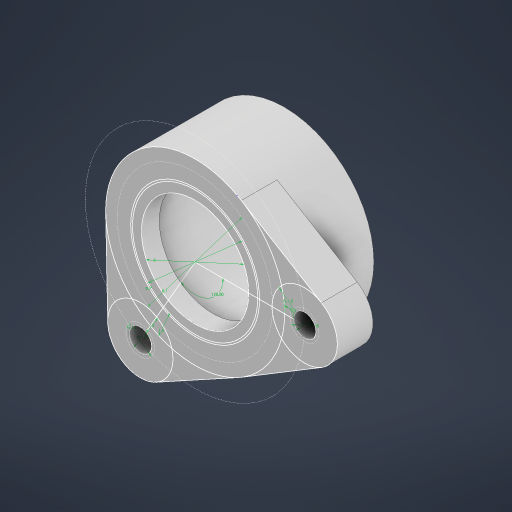
# Autodesk Inventor part: encoderauxiliary
Saved by Autodesk Inventor 2023.5 (Build 275446000, 446)
## iProperties
Created: 2024-12-07
Part Number: encoderauxiliary
Material: 一般
Document SubType Name: Modeling
Designer: IshiiLabHonda
Density: 1 g/cm^3
Appearance: 既定
Author: IshiiLabHonda
Autodesk Inventor part; units mm, degrees
ref_plane "YZ Plane" through (0, 0, 0) normal (1, 0, 0) x (0, 1, 0)
ref_plane "XZ Plane" through (0, 0, 0) normal (0, 1, 0) x (-1, 0, 0)
ref_plane "XY Plane" through (0, 0, 0) normal (0, 0, 1) x (1, 0, 0)
sketch "スケッチ1" plane through (0, 0, 0) normal (0, 0, 1) x (1, 0, 0)
  circle A0 centre (0, 0) radius 4.35 construction
  circle A1 centre (0, 0) radius 3.6
  circle A2 centre (0, 0) radius 5
  circle A3 centre (0, 0) radius 6.125 construction
  circle A4 centre (-3.0625, -5.3044) radius 0.625
  circle A5 centre (6.125, 0) radius 0.625
  circle A6 centre (-3.0625, -5.3044) radius 1.825
  circle A7 centre (6.125, 0) radius 1.825
  circle A8 centre (6.125, 0) radius 0.8 construction
  circle A9 centre (-3.0625, -5.3044) radius 0.8 construction
  line L0 (-4.9989, -0.1067) -> (-4.8871, -5.3434)
  line L1 (-2.1839, -6.904) -> (2.407, -4.3825)
  line L2 (2.5918, -4.2758) -> (7.071, -1.5607)
  line L3 (7.071, 1.5607) -> (2.5918, 4.2758)
  circle A10 centre (0, 0) radius 3
  line L4 (0, 0) -> (-3.0625, -5.3044)
  line L5 (0, 0) -> (6.125, 0)
  circle A11 centre (0, 0) radius 3.5
  point P0 (2.3702, 4.4025)
  dimension "d0" = 8.7
  dimension "d3" = 1.25
  dimension "d4" = 1.25
  dimension "d5" = 1.2
  dimension "d6" = 1.2
  dimension "d7" = 0.5
  dimension "d8" = 1.6
  dimension "d9" = 1.6
  dimension "d14" = 6
  dimension "d19" = 120
  dimension "d26" = 0.1
  dimension "d27" = 7
  dimension "d28" = 1.5
  constraints: 12 centre point, 12 end point, 11 coincident, 11 point on circle, 8 tangent, 1 horizontal
  measures "d0" diameter of A0
  measures "d3" diameter of A4
  measures "d4" diameter of A5
  measures "d5" radial gap between concentric circles of A4 A6
  measures "d6" radial gap between concentric circles of A7 A5
  measures "d8" diameter of A8
  measures "d9" diameter of A9
  measures "d14" diameter of A10
  measures "d19" angle of L5 L4
  measures "d26" radial gap between concentric circles of A1 A11
  measures "d27" diameter of A11
  measures "d28" radial gap between concentric circles of A2 A11
extrude "押し出し1" add sketch "スケッチ1" against normal blind 5 contours L5 A7 A2 A6 L4 A1 | A1 L4 A6 A2 A7 L5 | L5 A2 A7 | A7 A2 L5 | L4 A2 A6 | A6 A2 L4
extrude "押し出し2" add sketch "スケッチ1" against normal blind 1 contours L5 A11 L4 A1 | A1 L4 A11 L5 | A11 L4 A10 L5 | L5 A10 L4 A11
extrude "押し出し3" add sketch "スケッチ1" against normal blind 2 contours A7 A2 | A2 L3 A7 | A7 L2 A2 | A6 A2 | A2 L1 A6 | A6 L0 A2
equation "\"d3\" = d10"
equation "\"d4\" = d10"
equation "\"d6\" = d5"
equation "\"d8\" = d11"
equation "\"d9\" = d8"
equation "\"d10\" = 1.25"
equation "\"d11\" = 1.6"
